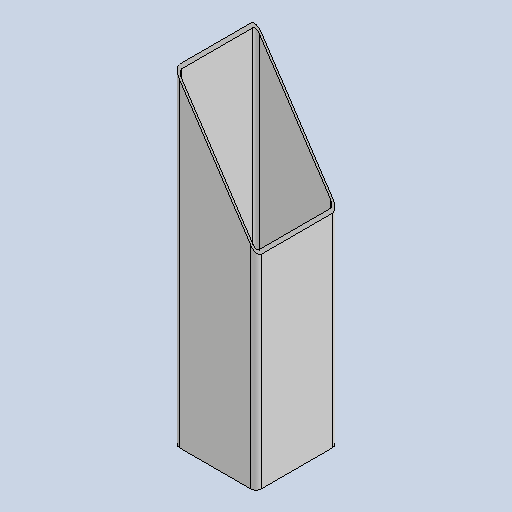
# Autodesk Inventor part: MSC 903 BASE TUBE
Saved by Autodesk Inventor 2025 (Build 290162010, 162A)
## iProperties
Created: 2024-07-01
Part Number: MSC 903 BASE TUBE
Material: Generic
Document SubType Name: Modeling
Designer: DELL
Density: 1 g/cm^3
Appearance: Default
Stock Number: МОО 903 базовая труба
Author: DELL
Autodesk Inventor part; units mm, degrees
ref_plane "YZ Plane" through (0, 0, 0) normal (1, 0, 0) x (0, 1, 0)
ref_plane "XZ Plane" through (0, 0, 0) normal (0, 1, 0) x (-1, 0, 0)
ref_plane "XY Plane" through (0, 0, 0) normal (0, 0, 1) x (1, 0, 0)
sketch "Sketch1" plane through (0, 0, 0) normal (0, 0, 1) x (1, 0, 0)
  line L0 (-35, 40) -> (35, 40)
  line L1 (40, 35) -> (40, -35)
  line L2 (35, -40) -> (-35, -40)
  line L3 (-40, -35) -> (-40, 35)
  line L4 (-40, 40) -> (40, -40) construction
  line L5 (40, 40) -> (-40, -40) construction
  arc A0 (-35, 40) -> (-40, 35) centre (-35, 35) ccw
  arc A1 (40, 35) -> (35, 40) centre (35, 35) ccw
  arc A2 (35, -40) -> (40, -35) centre (35, -35) ccw
  arc A3 (-40, -35) -> (-35, -40) centre (-35, -35) ccw
  line L6 (35, 38) -> (-35, 38)
  arc A4 (-35, 38) -> (-38, 35) centre (-35, 35) ccw
  line L7 (-38, 35) -> (-38, -35)
  arc A5 (-38, -35) -> (-35, -38) centre (-35, -35) ccw
  line L8 (-35, -38) -> (35, -38)
  arc A6 (35, -38) -> (38, -35) centre (35, -35) ccw
  line L9 (38, -35) -> (38, 35)
  arc A7 (38, 35) -> (35, 38) centre (35, 35) ccw
  point P0 (0, 0)
  dimension "d0" = 80
  dimension "d1" = 5
  dimension "d2" = 2
  constraints: 20 end point, 16 point on circle, 8 centre point, 8 point on line, 8 tangent, 4 parallel, 3 equal radius, 3 perpendicular, 2 midpoint, 1 horizontal, 7 other
  measures "d0" distance of L4.end L5.end
  measures "d1" radius of A0
  measures "d2" distance between parallel lines of L0 L6
extrude "Extrusion1" add sketch "Sketch1" along normal blind 320
sketch "Sketch2" plane through (0, 0, 0) normal (0, 1, 0) x (-1, 0, 0)
  line L0 (40, 0) -> (40, 320) projected
  line L1 (-40, 0) -> (-40, 320) projected
  line L2 (40, 320) -> (-40, 320)
  line L3 (40, 320) -> (-40, 198.8577)
  point P0 (0, 0)
  dimension "d5" = 123.44
  constraints: 4 end point, 1 horizontal, 1 point on line
  measures "d5" angle of L2 L3
extrude "Extrusion2" cut sketch "Sketch2" along normal through all both and the other way through all
body "Solid1"
